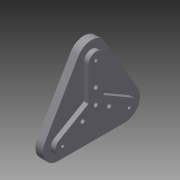
# Autodesk Inventor part: RibEnd
Saved by Autodesk Inventor 2015 (Build 190159000, 159)
## iProperties
Created: 2014-11-09
Part Number: RibEnd
Material: Generic
Document SubType Name: Modeling
Designer: Ryan
Density: 1 g/cm^3
Appearance: Default
Author: Ryan
Autodesk Inventor part; units mm, degrees
ref_plane "YZ Plane" through (0, 0, 0) normal (1, 0, 0) x (0, 1, 0)
ref_plane "XZ Plane" through (0, 0, 0) normal (0, 1, 0) x (-1, 0, 0)
ref_plane "XY Plane" through (0, 0, 0) normal (0, 0, 1) x (1, 0, 0)
sketch "Sketch1" plane through (0, 0, 0) normal (1, 0, 0) x (0, 1, 0)
  line L0 (2.9851, 0) -> (0, 0) construction
  line L1 (0, 0) -> (0, 4.2) construction
  circle A0 centre (0, 0) radius 1.425
  circle A1 centre (25.125, 0) radius 10
  circle A2 centre (-12.5625, 21.7589) radius 10
  circle A3 centre (-12.5625, -21.7589) radius 10
  line L2 (-7.5625, 30.4191) -> (30.125, 8.6603)
  line L3 (-22.5625, 21.7589) -> (-22.5625, -21.7589)
  line L4 (30.125, -8.6603) -> (-7.5625, -30.4191)
  line L5 (0, 0) -> (-12.5625, 21.7589) construction
  line L6 (-12.5625, 21.7589) -> (-12.5625, -21.7589) construction
  line L7 (-12.5625, 21.7589) -> (25.125, 0) construction
  line L8 (6.5, 3.5) -> (4.5, 3.5)
  line L9 (4.5, 3.5) -> (4.5, -3.5)
  line L10 (4.5, -3.5) -> (6.5, -3.5)
  line L11 (6.5, -3.5) -> (6.5, 3.5)
  line L12 (-4.5, 3.5) -> (-6.5, 3.5)
  line L13 (-6.5, 3.5) -> (-6.5, -3.5)
  line L14 (-6.5, -3.5) -> (-4.5, -3.5)
  line L15 (-4.5, -3.5) -> (-4.5, 3.5)
  dimension "d0" = 25.125
  dimension "d1" = 25.125
  dimension "d2" = 60
  dimension "d3" = 20
  dimension "d4" = 20
  dimension "d5" = 2.85
  dimension "d6" = 2
  dimension "d7" = 7
  dimension "d8" = 4.5
  constraints: 32 end point, 6 point on circle, 6 tangent, 4 centre point, 4 parallel, 3 horizontal, 2 perpendicular, 2 vertical, 1 coincident, 1 point on line, 1 symmetric about line, 6 other
  measures "d0" distance of L7.end L0.end
  measures "d1" distance of L5.start L5.end
  measures "d2" angle of L6 L7
  measures "d3" diameter of A1
  measures "d4" diameter of A3
  measures "d5" diameter of A0
  measures "d6" distance of L9.end L10.end
  measures "d7" distance of L10.end L8.start
  measures "d8" distance from line of L9 L0.end
extrude "Extrusion1" add sketch "Sketch1" against normal blind 5 contours A1 | A1 L4 A3 L3 A2 L2 | A2 | A3 | L11 L10 L9 L8 | L15 L14 L13 L12
sketch "Sketch6" plane through (0, 0, 0) normal (1, 0, 0) x (0, 0, -1)
  circle A0 centre (0, 25.125) radius 0.5
  circle A1 centre (-21.7589, -12.5625) radius 0.5
  circle A2 centre (21.7589, -12.5625) radius 0.5
  line L0 (0, 0) -> (0, 25.125)
  line L1 (0, 25.125) -> (-21.7589, -12.5625)
  line L2 (-21.7589, -12.5625) -> (21.7589, -12.5625)
  line L3 (21.7589, -12.5625) -> (0, 0)
  dimension "d32" = 25.125
  dimension "d33" = 25.125
  dimension "d34" = 60
  dimension "d35" = 1
  dimension "d36" = 1
  dimension "d37" = 1
  constraints: 8 end point, 3 centre point, 1 horizontal, 1 symmetric about line, 1 vertical
  measures "d32" distance of L2.end L0.start
  measures "d33" distance of L0.start L0.end
  measures "d34" angle of L2 L1
  measures "d35" diameter of A1
  measures "d36" diameter of A0
  measures "d37" diameter of A2
hole "Hole1" at (0, 25.125, 0) at (0, -12.5625, 21.7589) at (0, -12.5625, -21.7589) direction (-1, 0, 0) diameter 2 end through all
sketch "Sketch7" plane through (0, 0, 0) normal (1, 0, 0) x (0, 0, -1)
  circle A0 centre (0, 25.125) radius 5
  circle A1 centre (-21.7589, -12.5625) radius 1 projected
  circle A2 centre (-21.7589, -12.5625) radius 5
  circle A3 centre (21.7589, -12.5625) radius 5
  line L0 (-19.2589, -16.8926) -> (0, -5.7735)
  line L1 (0, -5.7735) -> (19.2589, -16.8926)
  line L2 (-24.2589, -8.2324) -> (-5, 2.8868)
  line L3 (5, 2.8868) -> (24.2589, -8.2324)
  line L4 (0, 0) -> (0, 25.125)
  line L5 (-21.7589, -12.5625) -> (0, 0)
  line L6 (21.7589, -12.5625) -> (0, 0)
  circle A4 centre (21.7589, -12.5625) radius 1 projected
  circle A5 centre (0, 25.125) radius 1 projected
  line L7 (-5, 25.125) -> (-5, 2.8868)
  line L8 (5, 2.8868) -> (5, 25.125)
  circle A6 centre (0, 0) radius 1.425
  dimension "d46" = 10
  constraints: 18 end point, 6 point on circle, 6 tangent, 5 parallel, 4 centre point, 3 point on line, 2 coincident, 2 concentric, 1 vertical
  measures "d46" diameter of A2
extrude "Extrusion6" add sketch "Sketch7" along normal blind 3
sketch "Sketch8" plane through (-5, 0, 0) normal (-1, 0, 0) x (0, 0, 1)
  line L0 (-3.5, 6.5) -> (3.5, 6.5)
  line L1 (3.5, 6.5) -> (3.5, 4.5)
  line L2 (3.5, 4.5) -> (-3.5, 4.5)
  line L3 (-3.5, 4.5) -> (-3.5, 6.5)
  line L4 (-3.5, -4.5) -> (3.5, -4.5)
  line L5 (3.5, -4.5) -> (3.5, -6.5)
  line L6 (3.5, -6.5) -> (-3.5, -6.5)
  line L7 (-3.5, -6.5) -> (-3.5, -4.5)
  circle A0 centre (0, 0) radius 1.425 projected
  line L8 (0, 1.3005) -> (0, 0) construction
  line L9 (0, 0) -> (-1.6567, 0) construction
  dimension "d49" = 7
  dimension "d50" = 2
  dimension "d51" = 4.5
  constraints: 20 end point, 4 parallel, 3 horizontal, 2 perpendicular, 1 point on line, 1 vertical, 5 other
  measures "d49" distance of L0.start L0.end
  measures "d50" distance of L2.end L0.start
  measures "d51" distance between parallel lines of L9 L2
extrude "Extrusion7" cut sketch "Sketch8" against normal blind 3 contours L0 L1 L2 L3 | L4 L5 L6 L7
sketch "Sketch9" plane through (3, 0, 0) normal (1, 0, 0) x (0, 0, -1)
  circle A0 centre (-8.6603, -5) radius 1.425
  circle A1 centre (8.6603, -5) radius 1.425
  circle A2 centre (0, 10) radius 1.425
  line L0 (0, 0) -> (0, 10)
  line L1 (0, 10) -> (-8.6603, -5)
  line L2 (-8.6603, -5) -> (8.6603, -5)
  circle A3 centre (0, 0) radius 1.425 projected
  line L3 (8.6603, -5) -> (0, 0)
  dimension "d54" = 10
  dimension "d55" = 10
  dimension "d56" = 60
  dimension "d57" = 2.85
  dimension "d58" = 2.85
  dimension "d59" = 2.85
  constraints: 8 end point, 3 centre point, 1 horizontal, 1 symmetric about line, 1 vertical
  measures "d54" distance of L0.start L0.end
  measures "d55" distance of L2.end L3.end
  measures "d56" angle of L2 L1
  measures "d57" diameter of A0
  measures "d58" diameter of A2
  measures "d59" diameter of A1
extrude "Extrusion8" cut sketch "Sketch9" against normal up to next contours L2 L1 A0 | A0 L1 L2 | L2 L3 A1 | A1 L3 L2 | L1 L0 A2 | A2 L0 L1
sketch "Sketch10" plane through (3, 0, 0) normal (1, 0, 0) x (0, 0, -1)
  circle A0 centre (0, 0) radius 1.425
  constraints: 1 centre point, 1 coincident
extrude "Extrusion9" cut sketch "Sketch10" against normal up to next
body "Solid1"
